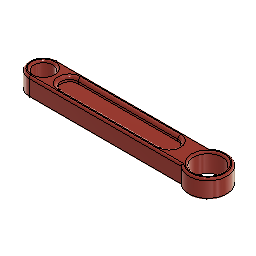
P2 - Pieza mecánica terminada (Autodesk Fusion 360 design; units mm, degrees)
Autodesk Fusion 360 part; units mm, degrees
mesh "Mesh1" [no effect]
sketch "Sketch1" plane through (0, 0, 0) normal (0, 0, 1) x (1, 0, 0)
  arc A0 (-89.1151, 15.0038) -> (-89.1132, -14.9962) centre (-89.1046, 0.0038) ccw
  line L0 (-89.1132, -14.9962) -> (70.8868, -14.9962)
  line L1 (-89.1132, -14.9962) -> (70.8868, -14.9962)
  circle A1 centre (84.114, 0) radius 14.9834
  circle A2 centre (84.114, 0) radius 15
  circle A3 centre (-89.1148, -0.0001) radius 10
  line L2 (-89.1132, -14.9962) -> (70.8868, -14.9962)
  arc A4 (70.8868, -14.9962) -> (70.8849, 15.0038) centre (84.1146, 0.0047) ccw
  line L3 (70.8849, 15.0038) -> (-89.1151, 15.0038)
  line L4 (70.8856, 15) -> (-89.1144, 15)
  dimension "d1" = 15
  dimension "d2" = 20
  dimension "d3" = 30
  dimension "d5" = 20
  dimension "d6" = 160
  dimension "d7" = 160
  constraint horizontal L0
  constraint horizontal L3
  constraint horizontal L4
  constraint coincident A0.end L0.start
  constraint coincident L0.end L1.end
  measures "d1" radius of A0
  measures "d2" diameter of A3
  measures "d3" diameter of A2
  measures "d5" radius of A4
  measures "d6" distance of A4.end A0.start
  measures "d7" distance of L0.end A0.end
sketch "Sketch2" plane through (0, 2.868, 10) normal (1, 0, 0) x (0, 1, 0)
  line L0 (12.1164, -1.68) -> (12.1164, -18.0338)
  arc A0 (10.1446, -0.0148) -> (12.1164, -1.68) centre (10.1446, -2.0148) cw
  line L1 (9.1421, -0.0148) -> (10.1446, -0.0148)
  arc A1 (6.1421, -3.0148) -> (9.1421, -0.0148) centre (9.1421, -3.0148) cw
  line L2 (6.1421, -5.0149) -> (6.1421, -3.0148)
  line L3 (-11.8579, -5.0148) -> (6.1421, -5.0149)
  line L4 (-11.868, -3.0001) -> (-11.8579, -5.0148)
  arc A2 (12.1164, -18.0338) -> (10.1165, -20.0148) centre (10.1165, -18.0148) cw
  line L5 (10.1165, -20.0148) -> (9.1164, -20.0148)
  arc A3 (9.1164, -20.0148) -> (6.1164, -17.0148) centre (9.1164, -17.0148) cw
  line L6 (6.1164, -17.0148) -> (6.1164, -15)
  line L7 (6.1164, -15) -> (-11.868, -15)
  line L8 (-11.868, -15) -> (-11.868, -17)
  arc A4 (-11.868, -17) -> (-14.868, -19.9985) centre (-14.8792, -16.9873) cw
  line L9 (-14.868, -19.9985) -> (-15.868, -20)
  arc A5 (-15.868, -20) -> (-17.8632, -17.9999) centre (-15.8404, -17.9772) cw
  line L10 (-17.8632, -17.9999) -> (-17.868, -2)
  arc A6 (-17.868, -2) -> (-15.8715, -0.0038) centre (-15.855, -2.0168) cw
  line L11 (-15.8715, -0.0038) -> (-14.868, 0)
  arc A7 (-14.868, 0) -> (-11.868, -3.0001) centre (-14.8864, -3.0183) cw
  dimension "d9" = 2
  dimension "d10" = 3
  dimension "d11" = 2
  dimension "d12" = 3
  dimension "d13" = 20
  dimension "d14" = 6
  dimension "d15" = 18
  dimension "d16" = 5
  constraint horizontal L3
  constraint horizontal L7
  constraint vertical L2
  constraint vertical L6
  constraint vertical L0
  constraint horizontal L1
  constraint horizontal L5
  constraint tangent A2 L5
  constraint tangent A3 L6
  constraint tangent A1 L2
  constraint tangent A0 L1
  constraint tangent L1 A1
  constraint tangent L5 A3
  measures "d9" radius of A0
  measures "d10" radius of A1
  measures "d11" radius of A2
  measures "d12" radius of A3
  measures "d13" distance of L1 L5
  measures "d14" distance of L0 L6
  measures "d15" distance of L2.start L3.start
  measures "d16" distance of L1 L3
extrude "Extrude1" add sketch "Sketch1" along normal mid plane 20 contours A0 L0 L1 L2 A4 L3
fillet "Fillet1" radius 2 10 edges at (-9.1151, 15.0038, 10) (-104.1046, 0.0028, 10) (-9.1132, -14.9962, 10) (-9.1132, -14.9962, -10) (-104.1046, 0.0028, -10) (-9.1151, 15.0038, -10) (104.1146, 0.006, 10) (104.1146, 0.006, -10) (70.1291, 5.4242, 10) (-98.4381, 3.6161, 10)
sketch "Sketch3" plane through (0, 0, 6) normal (0, 0, 1) x (1, 0, 0)
  line L0 (-61.6299, -8.959) -> (43.3701, -8.9552)
  arc A0 (43.3701, -8.9552) -> (43.3694, 9.0448) centre (43.3697, 0.0448) ccw
  line L1 (43.3694, 9.0448) -> (-61.6306, 9.041)
  arc A1 (-61.6306, 9.041) -> (-61.6299, -8.959) centre (-61.6303, 0.041) ccw
  line L2 (-70.6303, 0.0407) -> (52.3697, 0.0451) construction
  dimension "d20" = 18
  dimension "d21" = 105
  constraint tangent L0 A0
  constraint tangent A0 L1
  constraint parallel L0 L1
  constraint tangent L1 A1
  constraint tangent L0 A1
  constraint midpoint A1 L2.start
  constraint midpoint A0 L2.end
  measures "d20" distance of L0 L1
  measures "d21" horizontal distance of A1.centre A0.centre
extrude "Extrude2" cut sketch "Sketch3" against normal blind 5 from surface at 4
mirror "Mirror1" about plane through (0, 0, 0) normal (0, 0, 1) of "Extrude2"
fillet "Fillet2" radius 3 8 edges at (-9.1306, 9.0429, 10) (52.3697, 0.0451, 10) (-9.1299, -8.9571, 10) (-70.6303, 0.0407, 10) (-9.1306, 9.0429, -10) (-70.6303, 0.0407, -10) (-9.1299, -8.9571, -10) (52.3697, 0.0451, -10)
